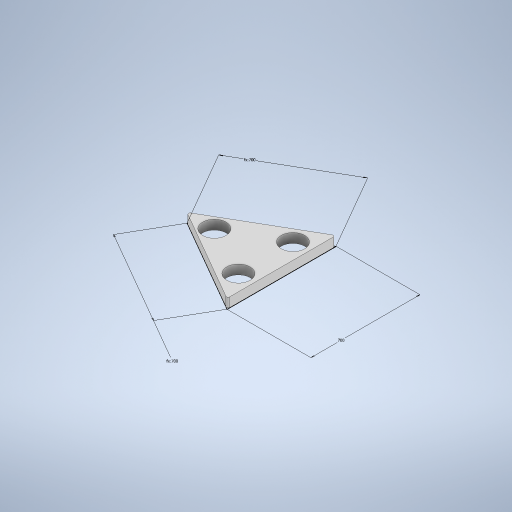
# Autodesk Inventor part: BELLY
Saved by Autodesk Inventor 2023.2 (Build 272271000, 271)
## iProperties
Created: 2023-10-07
Part Number: BELLY
Material: Generic
Document SubType Name: Modeling
Designer: 271663e
Density: 1 g/cm^3
Appearance: Default
Author: 271663e
Autodesk Inventor part; units mm, degrees
ref_plane "YZ Plane" through (0, 0, 0) normal (1, 0, 0) x (0, 1, 0)
ref_plane "XZ Plane" through (0, 0, 0) normal (0, 1, 0) x (-1, 0, 0)
ref_plane "XY Plane" through (0, 0, 0) normal (0, 0, 1) x (1, 0, 0)
sketch "Sketch1" plane through (0, 0, 0) normal (0, 1, 0) x (-1, 0, 0)
  line L0 (0.2037, 0) -> (0, 0)
  line L1 (0, 0) -> (-606.2178, 350)
  line L2 (-606.2178, 350) -> (-606.2178, -350)
  line L3 (-606.2178, -350) -> (0, 0)
  point P0 (-178.8272, 3.3733)
  point P1 (-505.1815, 175)
  point P2 (-505.1815, -175)
  dimension "d0" = 700
  dimension "d1" = 700
  dimension "d2" = 700
  constraints: 8 end point, 1 horizontal, 1 perpendicular
  measures "d0" distance of L0.end L1.end
  measures "d1" distance of L2.end L0.end
  measures "d2" distance of L1.end L2.end
extrude "Extrusion1" add sketch "Sketch1" along normal blind 60
hole "Hole3" at (505.1815, 0, -175) at (178.8272, 0, 3.3733) at (505.1815, 0, 175) direction (0, 1, 0) diameter 150 end through all
fillet "Fillet1" radius 10 1 edges at (0, 30, 0)
fillet "Fillet2" radius 10 1 edges at (606.2178, 30, 350)
fillet "Fillet3" radius 10 1 edges at (606.2178, 30, -350)
equation "\"d0\" = d1"
equation "\"d1\" = d2"
body "Solid1"
